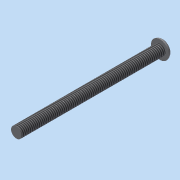
# Autodesk Inventor part: m3x40
Saved by Autodesk Inventor 2015 (Build 190159000, 159)
## iProperties
Created: 2016-09-08
Part Number: m3x40
Material: Generic
Document SubType Name: Modeling
Designer: Dustin
Density: 1 g/cm^3
Appearance: Default
Author: Dustin
Autodesk Inventor part; units mm, degrees
ref_plane "YZ Plane" through (0, 0, 0) normal (1, 0, 0) x (0, 1, 0)
ref_plane "XZ Plane" through (0, 0, 0) normal (0, 1, 0) x (-1, 0, 0)
ref_plane "XY Plane" through (0, 0, 0) normal (0, 0, 1) x (1, 0, 0)
sketch "Sketch1" plane through (0, 0, 0) normal (0, 0, 1) x (1, 0, 0)
  line L0 (0, 0) -> (1.5, 0)
  line L1 (1.5, 0) -> (1.5, 40)
  line L2 (1.5, 40) -> (0, 40)
  line L3 (0, 40) -> (0, 0)
  line L4 (0, 40) -> (2.5, 40)
  line L5 (2.5, 40) -> (2.5, 41)
  line L6 (2.5, 41) -> (0, 41)
  line L7 (0, 41) -> (0, 40)
  dimension "d0" = 1.5
  dimension "d1" = 2.5
  dimension "d2" = 1
  dimension "d7" = 40
  constraints: 16 end point, 4 parallel, 2 horizontal, 2 perpendicular
  measures "d0" distance of L0.start L0.end
  measures "d1" distance of L5.end L6.end
  measures "d2" distance of L4.end L5.end
  measures "d7" distance of L2.end L0.start
revolve "Revolution1" add sketch "Sketch1" angle 360 about axis through (0, 40, 0) along (0, -1, 0)
fillet "Fillet1" radius 1 1 edges at (-2.5, 41, 0)
thread "Thread1" size "M3x0.5" class "6g" standard "ANSI Metric M Profile" full length
body "Solid1"
